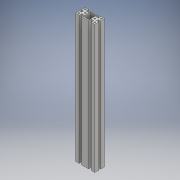
# Autodesk Inventor part: 3060400
Saved by Autodesk Inventor 2018 (Build 220112000, 112)
## iProperties
Created: 2020-09-14
Part Number: 3060400
Material: 일반
Document SubType Name: Sheet Metal
Designer: j3jjj
Density: 1 g/cm^3
Sheet Metal Rule: 기본값_mm
Appearance: 기본값
Author: j3jjj
Autodesk Inventor part; units mm, degrees
ref_plane "YZ Plane" through (0, 0, 0) normal (1, 0, 0) x (0, 1, 0)
ref_plane "XZ Plane" through (0, 0, 0) normal (0, 1, 0) x (-1, 0, 0)
ref_plane "XY Plane" through (0, 0, 0) normal (0, 0, 1) x (1, 0, 0)
sketch "스케치2" plane through (0, 0, 0) normal (0, 1, 0) x (-1, 0, 0)
  point P0 (0, 0)
sketch "스케치3" plane through (0, 0, 0) normal (0, 0, 1) x (1, 0, 0)
  line L0 (9, 12) -> (-9, 12)
  line L1 (-9, 12) -> (-9, -12)
  line L2 (-9, -12) -> (9, -12)
  circle A0 centre (-15, 0) radius 2.5
  line L3 (-30, 3) -> (-23.0102, 3)
  line L4 (-23.0102, 3) -> (-23.0102, -3)
  line L5 (-23.0102, -3) -> (-30, -3)
  circle A1 centre (-25, 10) radius 2.5
  circle A2 centre (-25, -10) radius 2.5
  line L6 (-11, 15) -> (-11, 7)
  line L7 (-11, 7) -> (-19, 7)
  line L8 (-19, 7) -> (-19, 15)
  line L9 (-11, -15) -> (-11, -7)
  line L10 (-11, -7) -> (-19, -7)
  line L11 (-19, -7) -> (-19, -15)
  line L12 (0, 0) -> (0, 6.2696)
  line L13 (-9, 12) -> (9, 12)
  line L14 (9, 12) -> (9, -12)
  line L15 (9, -12) -> (-9, -12)
  circle A3 centre (15, 0) radius 2.5
  line L16 (30, 3) -> (23.0102, 3)
  line L17 (23.0102, 3) -> (23.0102, -3)
  line L18 (23.0102, -3) -> (30, -3)
  circle A4 centre (25, 10) radius 2.5
  circle A5 centre (25, -10) radius 2.5
  line L19 (11, 15) -> (11, 7)
  line L20 (11, 7) -> (19, 7)
  line L21 (19, 7) -> (19, 15)
  line L22 (11, -15) -> (11, -7)
  line L23 (11, -7) -> (19, -7)
  line L24 (19, -7) -> (19, -15)
  line L25 (-30, 15) -> (-30, 3)
  line L26 (-30, -3) -> (-30, -15)
  line L27 (-30, -15) -> (-19, -15)
  line L28 (-11, -15) -> (11, -15)
  line L29 (19, -15) -> (30, -15)
  line L30 (30, -15) -> (30, -3)
  line L31 (30, 3) -> (30, 15)
  line L32 (30, 15) -> (19, 15)
  line L33 (11, 15) -> (-11, 15)
  line L34 (-19, 15) -> (-30, 15)
  line L35 (-9, 12) -> (-9, -12)
  line L36 (9, -12) -> (9, 12)
  line L37 (9, 12) -> (-9, 12)
  line L38 (-9, -12) -> (9, -12)
  dimension "d31" = 24
  dimension "d32" = 12
  dimension "d35" = 15
  dimension "d36" = 9
  dimension "d37" = 5
  dimension "d38" = 5
  dimension "d39" = 20
  dimension "d40" = 10
  dimension "d41" = 25
  dimension "d42" = 5
  dimension "d45" = 4
  dimension "d46" = 8
  dimension "d51" = 14.0102
  dimension "d55" = 6
  dimension "d56" = 3
  dimension "d58" = 60
  dimension "d59" = 30
  dimension "d60" = 15
  dimension "d61" = 8
  dimension "d62" = 8
  dimension "d63" = 8
  dimension "d64" = 14
  dimension "d65" = 7
  dimension "d66" = 19
  dimension "d67" = 15
  dimension "d68" = 60
  dimension "d69" = 6
  constraints: 78 end point, 19 symmetric about line, 6 centre point, 6 parallel, 5 horizontal, 4 collinear, 4 point on line, 4 vertical, 3 perpendicular, 3 other
  measures "d31" distance between parallel lines of L2 L0
  measures "d32" distance from line of L12.start L0
  measures "d35" distance of L12.start A0.centre
  measures "d36" distance from line of L12.start L1
  measures "d37" diameter of A1
  measures "d38" diameter of A2
  measures "d39" distance of A2.centre A1.centre
  measures "d40" vertical distance of L12.start A1.centre
  measures "d41" horizontal distance of L12.start A1.centre
  measures "d42" diameter of A0
  measures "d45" distance from line of A0.centre L11
  measures "d46" distance between parallel lines of L9 L11
  measures "d51" distance between parallel lines of L1 L4
  measures "d55" distance between parallel lines of L5 L3
  measures "d56" distance from line of A0.centre L3
  measures "d58" distance between parallel lines of L31 L25
  measures "d59" distance between parallel lines of L27 L34
  measures "d60" distance from line of L12.start L34
  measures "d61" distance between parallel lines of L6 L8
  measures "d62" distance of L10.end L11.end
  measures "d63" distance of L9.start L9.end
  measures "d64" distance between parallel lines of L7 L10
  measures "d65" distance from line of L12.start L7
  measures "d66" distance between parallel lines of L12 L8
  measures "d67" distance from line of L12.start L33
  measures "d68" distance between parallel lines of L26 L30
  measures "d69" distance from line of L24 A5.centre
extrude "돌출2" add sketch "스케치3" along normal blind 400
equation "\"TransitionRadius\" = BendRadius"
equation "\"BendRadius\" = 0.5"
